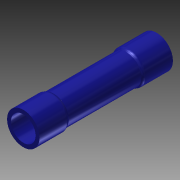
# Autodesk Inventor part: point 107 double sided femal tube blue
Saved by Autodesk Inventor 2014 (Build 180170000, 170)
## iProperties
Created: 2013-07-20
Part Number: point 107 double sided femal tube blue
Material: Generic
Document SubType Name: Modeling
Designer: Saville
Mass: 0.388943 g
Surface Area: 11.3426 cm^2
Volume: 0.388943 cm^3
Density: 1 g/cm^3
Appearance: Default
Author: Saville
Autodesk Inventor part; units mm, degrees
ref_plane "YZ Plane" through (0, 0, 0) normal (1, 0, 0) x (0, 1, 0)
ref_plane "XZ Plane" through (0, 0, 0) normal (0, 1, 0) x (-1, 0, 0)
ref_plane "XY Plane" through (0, 0, 0) normal (0, 0, 1) x (1, 0, 0)
sketch "Sketch1" plane through (0, 0, 0) normal (0, 0, 1) x (1, 0, 0)
  circle A0 centre (0, 0) radius 2.7559
  dimension "d0" = 5.5118
  constraints: 1 centre point, 1 coincident
  measures "d0" diameter of A0
extrude "Extrusion1" add sketch "Sketch1" along normal mid plane 24.7269
sketch "Sketch2" plane through (0, 0, 12.36345) normal (0, 0, 1) x (1, 0, 0)
  circle A0 centre (0, 0) radius 2.7559 projected
  circle A1 centre (0, 0) radius 3.0099
  dimension "d3" = 6.0198
  constraints: 1 centre point, 1 coincident
  measures "d3" diameter of A1
extrude "Extrusion2" add sketch "Sketch2" against normal blind 5.461
fillet "Fillet1" radius 0.254 1 edges at (-2.7559, 0, 6.9024)
fillet "Fillet2" radius 0.762 2 edges at (-3.0098, 0, 6.9024) (-3.0099, 0, 6.9024)
mirror "Mirror1" about plane through (0, 0, 0) normal (0, 0, 1) of "Extrusion2", "Fillet1", "Fillet2"
shell "Shell1" thickness 0.7239 removed faces 2 at (0.974146, -1.090517, -12.36345) at (0.974146, -1.090517, 12.36345)
sketch "Sketch3" plane through (0, 0, 0) normal (1, 0, 0) x (0, 1, 0)
  arc A0 (-3.0099, 7.320471) -> (-2.8194, 6.816455) centre (-2.2479, 7.320471) ccw
  line L0 (-3.0099, 7.320471) -> (-3.0099, 12.36345)
  line L1 (-3.0099, 12.36345) -> (-2.286, 12.36345)
  line L2 (-2.286, 12.36345) -> (-2.286, 7.320471)
  arc A1 (-2.286, 7.320471) -> (-2.276475, 7.29527) centre (-2.2479, 7.320471) ccw
  arc A2 (-2.032, 6.64845) -> (-2.276475, 7.29527) centre (-3.0099, 6.64845) ccw
  line L3 (-2.032, 6.64845) -> (-2.032, -6.64845)
  arc A3 (-2.276475, -7.29527) -> (-2.032, -6.64845) centre (-3.0099, -6.64845) ccw
  arc A4 (-2.276475, -7.29527) -> (-2.286, -7.320471) centre (-2.2479, -7.320471) ccw
  line L4 (-2.286, -7.320471) -> (-2.286, -12.36345)
  line L5 (-2.286, -12.36345) -> (-3.0099, -12.36345)
  line L6 (-3.0099, -12.36345) -> (-3.0099, -7.320471)
  arc A5 (-2.8194, -6.816455) -> (-3.0099, -7.320471) centre (-2.2479, -7.320471) ccw
  arc A6 (-2.8194, -6.816455) -> (-2.7559, -6.64845) centre (-3.0099, -6.64845) ccw
  line L7 (-2.7559, -6.64845) -> (-2.7559, 6.64845)
  arc A7 (-2.7559, 6.64845) -> (-2.8194, 6.816455) centre (-3.0099, 6.64845) ccw
  arc A8 (2.8194, 6.816455) -> (3.0099, 7.320471) centre (2.2479, 7.320471) ccw
  arc A9 (2.8194, 6.816455) -> (2.7559, 6.64845) centre (3.0099, 6.64845) ccw
  line L8 (2.7559, 6.64845) -> (2.7559, -6.64845)
  arc A10 (2.7559, -6.64845) -> (2.8194, -6.816455) centre (3.0099, -6.64845) ccw
  arc A11 (3.0099, -7.320471) -> (2.8194, -6.816455) centre (2.2479, -7.320471) ccw
  line L9 (3.0099, -7.320471) -> (3.0099, -12.36345)
  line L10 (3.0099, -12.36345) -> (2.286, -12.36345)
  line L11 (2.286, -12.36345) -> (2.286, -7.320471)
  arc A12 (2.286, -7.320471) -> (2.276475, -7.29527) centre (2.2479, -7.320471) ccw
  arc A13 (2.032, -6.64845) -> (2.276475, -7.29527) centre (3.0099, -6.64845) ccw
  line L12 (2.032, -6.64845) -> (2.032, 6.64845)
  arc A14 (2.276475, 7.29527) -> (2.032, 6.64845) centre (3.0099, 6.64845) ccw
  arc A15 (2.276475, 7.29527) -> (2.286, 7.320471) centre (2.2479, 7.320471) ccw
  line L13 (2.286, 7.320471) -> (2.286, 12.36345)
  line L14 (2.286, 12.36345) -> (3.0099, 12.36345)
  line L15 (3.0099, 12.36345) -> (3.0099, 7.320471)
  line L16 (-2.032, -7.41045) -> (-1.3589, -7.41045)
  line L17 (-1.3589, -7.41045) -> (-1.3589, 7.41045)
  line L18 (-1.3589, 7.41045) -> (-2.032, 7.41045)
  line L19 (-2.032, 7.41045) -> (-2.032, -7.41045)
  line L20 (0, -17.30883) -> (0, 17.30883)
  point P0 (0, 0)
  dimension "d9" = 0.6731
  dimension "d10" = 0.762
  dimension "d11" = 0.762
  constraints: 8 end point, 2 parallel, 1 collinear, 1 horizontal, 1 perpendicular
  measures "d9" distance between parallel lines of L17 L19
  measures "d10" distance from line of L3.end L16
  measures "d11" distance from line of L18 L3.start
revolve "Revolution1" add sketch "Sketch3" angle 360 about axis through (0, 0, -10) along (0, 0, 1) separate body contours L19 L18 L17 L16 L3
chamfer "Chamfer1" distance 0.2032 angle 45 2 edges at (0, 1.3589, 7.4105) (0, 1.3589, -7.4105)
body "Solid1"
body "Solid2"
